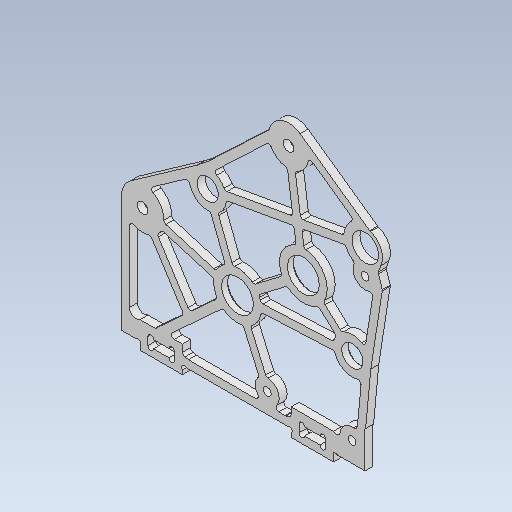
# Autodesk Inventor part: アームフレーム改二
Saved by Autodesk Inventor 2020.2 (Build 242310000, 310)
## iProperties
Created: 2020-02-29
Part Number: アームフレーム改二
Material: アルミニウム 2014-T4
Document SubType Name: Modeling
Designer: aoyam
Density: 2.8 g/cm^3
Appearance: サテン
Mass: 22.4919 g
Surface Area: 98.9037 cm^2
Volume: 8.03281 cm^3
Author: aoyam
Autodesk Inventor part; units mm, degrees
ref_plane "YZ Plane" through (0, 0, 0) normal (1, 0, 0) x (0, 1, 0)
ref_plane "XZ Plane" through (0, 0, 0) normal (0, 1, 0) x (-1, 0, 0)
ref_plane "XY Plane" through (0, 0, 0) normal (0, 0, 1) x (1, 0, 0)
sketch "ギア線図" plane through (0, 0, 0) normal (0, 0, 1) x (1, 0, 0)
  circle A0 centre (11.2246, -29.111) radius 11.1
  circle A1 centre (54.569, -27.2294) radius 20.05
  circle A2 centre (54.569, -27.2294) radius 4
  circle A3 centre (36.0807, -10.2532) radius 11.1
  circle A4 centre (39.569, -43.72) radius 2.05
  circle A5 centre (69.569, -43.72) radius 2.05
  circle A6 centre (72.4026, -13.8541) radius 2.05
  circle A7 centre (39.569, -43.72) radius 15
  circle A8 centre (69.569, -43.72) radius 15
  circle A9 centre (72.4026, -13.8541) radius 15
  circle A10 centre (54.569, -27.2294) radius 5.5 construction
  circle A11 centre (11.2246, -29.111) radius 13 construction
  circle A12 centre (54.569, -27.2294) radius 20.5 construction
  circle A13 centre (36.0807, -10.2532) radius 20.55
  circle A14 centre (36.0807, -10.2532) radius 21.5 construction
  circle A15 centre (36.0807, -10.2532) radius 13 construction
  circle A16 centre (39.569, -43.72) radius 2.5 construction
  circle A17 centre (69.569, -43.72) radius 2.5 construction
  circle A18 centre (72.4026, -13.8541) radius 2.5 construction
  circle A19 centre (11.2246, -29.111) radius 20.1
  circle A20 centre (11.2246, -29.111) radius 22 construction
  line L0 (39.569, -43.72) -> (69.569, -43.72)
  circle A21 centre (0, 0) radius 20.1
  circle A22 centre (0, 0) radius 22 construction
  circle A23 centre (39.569, -43.72) radius 9.5 construction
  circle A24 centre (69.569, -43.72) radius 9.5 construction
  circle A25 centre (72.4026, -13.8541) radius 9.5 construction
  line L1 (39.569, -43.72) -> (33.651, -38.3369)
  line L2 (39.569, -43.72) -> (54.569, -27.2294)
  circle A26 centre (33.651, -38.3369) radius 2.25
  circle A27 centre (54.569, -27.2294) radius 4.55
  line L3 (39.569, -43.72) -> (45.487, -49.103)
  circle A28 centre (45.487, -49.103) radius 1.3
  line L4 (69.569, -43.72) -> (54.569, -27.2294)
  line L5 (54.569, -27.2294) -> (72.4026, -13.8541)
  line L6 (69.569, -43.72) -> (75.487, -38.3369)
  line L7 (69.569, -43.72) -> (63.651, -49.103)
  circle A29 centre (63.651, -49.103) radius 1.3
  circle A30 centre (75.487, -38.3369) radius 1.3
  line L8 (39.569, -43.72) -> (11.2246, -29.111)
  line L9 (77.2027, -20.2541) -> (72.4026, -13.8541)
  circle A31 centre (77.2027, -20.2541) radius 1.3
  circle A32 centre (67.6026, -7.4541) radius 1.3
  point P0 (58.2233, -20.0465)
  point P1 (42.0436, -35)
  point P2 (21.5995, 15.2696)
  point P3 (38.2329, 5.9161)
  point P4 (24.1755, 8.4229)
  point P5 (21.6039, 15.1272)
  point P6 (23.3458, 16.3469)
  point P7 (23.3177, 16.3886)
  dimension "d7" = 22.2
  dimension "d8" = 40.1
  dimension "d9" = 8
  dimension "d11" = 22.2
  dimension "d12" = 4.1
  dimension "d13" = 4.1
  dimension "d14" = 4.1
  dimension "d15" = 30
  dimension "d16" = 30
  dimension "d17" = 30
  dimension "d18" = 11
  dimension "d21" = 26
  dimension "d29" = 41
  dimension "d39" = 22.2921
  dimension "d40" = 22.2921
  dimension "d41" = 22.2921
  dimension "d43" = 41.1
  dimension "d44" = 43
  dimension "d45" = 26
  dimension "d46" = 5
  dimension "d47" = 5
  dimension "d48" = 5
  dimension "d49" = 40.2
  dimension "d50" = 44
  dimension "d53" = 40.2
  dimension "d55" = 44
  dimension "d58" = 19
  dimension "d59" = 19
  dimension "d60" = 19
  dimension "d86" = 8
  dimension "d87" = 4.5
  dimension "d121" = 8
  dimension "d122" = 2.6
  dimension "d123" = 8
  dimension "d124" = 8
  dimension "d125" = 2.6
  dimension "d126" = 2.6
  dimension "d127" = 31.8878
  dimension "d128" = 8
  dimension "d129" = 2.6
  constraints: 33 centre point, 20 coincident, 20 end point, 7 tangent, 5 perpendicular, 3 concentric, 2 horizontal, 1 symmetric about line, 2 other
  measures "d7" diameter of A0
  measures "d8" diameter of A1
  measures "d9" diameter of A2
  measures "d11" diameter of A3
  measures "d12" diameter of A4
  measures "d13" diameter of A5
  measures "d14" diameter of A6
  measures "d15" diameter of A7
  measures "d16" diameter of A8
  measures "d17" diameter of A9
  measures "d18" diameter of A10
  measures "d21" diameter of A11
  measures "d29" diameter of A12
  measures "d39" distance of A4.centre A1.centre
  measures "d40" distance of A5.centre A1.centre
  measures "d41" distance of A6.centre A1.centre
  measures "d43" diameter of A13
  measures "d44" diameter of A14
  measures "d45" diameter of A15
  measures "d46" diameter of A16
  measures "d47" diameter of A17
  measures "d48" diameter of A18
  measures "d49" diameter of A19
  measures "d50" diameter of A20
  measures "d53" diameter of A21
  measures "d55" diameter of A22
  measures "d58" diameter of A23
  measures "d59" diameter of A24
  measures "d60" diameter of A25
  measures "d86" distance of L1.start L1.end
  measures "d87" diameter of A26
  measures "d121" distance of L1.start L3.end
  measures "d122" diameter of A28
  measures "d123" distance of L4.start L6.end
  measures "d124" distance of L7.start L7.end
  measures "d125" diameter of A29
  measures "d126" diameter of A30
  measures "d127" distance of L1.start L8.end
  measures "d128" distance of L9.start L5.end
  measures "d129" diameter of A31
sketch "スケッチ3" plane through (0, 0, 0) normal (0, 0, 1) x (1, 0, 0)
  circle A0 centre (54.569, -27.2294) radius 20.05 construction
  circle A1 centre (39.569, -43.72) radius 2.05 construction
  circle A2 centre (69.569, -43.72) radius 2.05 construction
  circle A3 centre (72.4026, -13.8541) radius 2.05 construction
  circle A4 centre (39.569, -43.72) radius 15 construction
  circle A5 centre (69.569, -43.72) radius 15 construction
  circle A6 centre (72.4026, -13.8541) radius 15 construction
  line L0 (39.569, -43.72) -> (45.487, -49.103)
  line L1 (45.487, -49.103) -> (39.569, -43.72)
  line L2 (39.569, -43.72) -> (33.651, -38.3369)
  line L3 (39.569, -43.72) -> (41.0777, -42.0614)
  circle A7 centre (33.651, -38.3369) radius 1.3
  circle A8 centre (45.487, -49.103) radius 1.3
  line L4 (69.569, -43.72) -> (68.0603, -42.0614)
  line L5 (69.569, -43.72) -> (75.487, -38.3369)
  line L6 (69.569, -43.72) -> (63.651, -49.103)
  circle A9 centre (63.651, -49.103) radius 1.3
  circle A10 centre (75.487, -38.3369) radius 1.3
  line L7 (72.4026, -13.8541) -> (70.609, -15.1993)
  line L8 (67.6026, -7.4541) -> (72.4026, -13.8541)
  line L9 (72.4026, -13.8541) -> (77.2027, -20.2541)
  circle A11 centre (67.6026, -7.4541) radius 1.3
  circle A12 centre (77.2027, -20.2541) radius 1.3
  circle A13 centre (39.569, -43.72) radius 5
  circle A14 centre (69.569, -43.72) radius 5
  circle A15 centre (72.4026, -13.8541) radius 5
  circle A16 centre (54.569, -27.2294) radius 4
  circle A17 centre (36.0807, -10.2532) radius 11.1 construction
  line L10 (87.4026, -58.72) -> (21.3486, -58.72)
  line L11 (87.4026, 3.1749) -> (87.4026, -58.72)
  circle A18 centre (36.0807, -10.2532) radius 6
  circle A19 centre (23.1948, 12.8161) radius 1.5
  circle A20 centre (59.3303, 1.1874) radius 1.5
  circle A21 centre (11.2246, -29.111) radius 6
  circle A22 centre (14.4482, -54.9706) radius 1.5
  line L12 (87.4026, 3.1749) -> (31.1389, 3.1749)
  line L13 (31.1389, 3.1749) -> (25.7575, 16.2256)
  line L14 (26.6296, -46.3454) -> (10.2913, -53.0824)
  line L15 (10.2913, -53.0824) -> (10.2913, -58.72)
  line L16 (10.2913, -58.72) -> (21.3486, -58.72)
  line L17 (26.6296, -46.3454) -> (26.6296, -10.2532)
  line L18 (26.6296, -10.2532) -> (18.7982, 13.9762)
  line L19 (18.7982, 13.9762) -> (25.7575, 16.2256)
  circle A23 centre (36.0807, -10.2532) radius 13 projected
  circle A24 centre (36.0807, -10.2532) radius 14
  circle A25 centre (36.0807, -10.2532) radius 17
  line L20 (50.0807, -10.2532) -> (50.0807, 3.1749)
  line L21 (26.6296, -24.2532) -> (36.0807, -24.2532)
  circle A26 centre (33.651, -38.3369) radius 2
  point P0 (0, 0)
  point P1 (0, 0)
  point P2 (30.1122, 5.6646)
  point P3 (23.0867, 0.7083)
  point P4 (26.6296, -24.3839)
  point P5 (46.5059, 3.1749)
  point P6 (40.0412, 3.1749)
  point P7 (26.6296, -20.5817)
  dimension "d61" = 8
  dimension "d62" = 8
  dimension "d63" = 2.6
  dimension "d64" = 2.6
  dimension "d65" = 8
  dimension "d66" = 8
  dimension "d67" = 2.6
  dimension "d68" = 2.6
  dimension "d69" = 8
  dimension "d70" = 8
  dimension "d71" = 2.6
  dimension "d72" = 2.6
  dimension "d73" = 10
  dimension "d74" = 10
  dimension "d75" = 10
  dimension "d76" = 8
  dimension "d79" = 12
  dimension "d82" = 26
  dimension "d83" = 1
  dimension "d84" = 3
  dimension "d85" = 4
  dimension "d98" = 12
  constraints: 44 end point, 18 centre point, 13 coincident, 8 perpendicular, 5 point on circle, 3 horizontal, 3 line through centre, 3 point on line, 2 collinear, 2 tangent, 2 vertical
  measures "d61" distance of L0.start L0.end
  measures "d62" distance of L0.start L2.end
  measures "d63" diameter of A7
  measures "d64" diameter of A8
  measures "d65" distance of L4.start L5.end
  measures "d66" distance of L4.start L6.end
  measures "d67" diameter of A9
  measures "d68" diameter of A10
  measures "d69" distance of L8.start L8.end
  measures "d70" distance of L8.end L9.end
  measures "d71" diameter of A11
  measures "d72" diameter of A12
  measures "d73" diameter of A13
  measures "d74" diameter of A14
  measures "d75" diameter of A15
  measures "d76" diameter of A16
  measures "d79" diameter of A18
  measures "d82" diameter of A23
  measures "d83" radial gap between concentric circles of A23 A24
  measures "d84" radial gap between concentric circles of A24 A25
  measures "d85" diameter of A26
  measures "d98" diameter of A21
sketch "スケッチ6" plane through (0, 0, 0) normal (0, 0, 1) x (1, 0, 0)
  circle A0 centre (36.0807, -10.2532) radius 6 projected
  circle A1 centre (11.2246, -29.111) radius 6 projected
  circle A2 centre (54.569, -27.2294) radius 4 projected
  circle A3 centre (14.4482, -54.9706) radius 1.5 projected
  circle A4 centre (59.3303, 1.1874) radius 1.5 projected
  line L0 (-26.5518, -24.6836) -> (-26.5518, -65.4706)
  line L1 (-26.5518, -65.4706) -> (62.634, -65.4706)
  line L2 (62.7829, 5.6168) -> (32.1759, 5.6168)
  line L3 (-26.5518, -24.6836) -> (-26.5518, 11.7202)
  line L4 (-26.5518, 11.7202) -> (32.1759, 5.6168)
  circle A5 centre (9.9716, -0.138) radius 1.5
  line L5 (14.4482, -54.9706) -> (22.4482, -54.9706)
  circle A6 centre (22.4482, -54.9706) radius 1.5
  circle A7 centre (0, 0) radius 4.025
  circle A8 centre (0, 0) radius 6.025
  circle A9 centre (54.4482, -54.9706) radius 1.5
  circle A10 centre (39.569, -43.72) radius 15 projected
  circle A11 centre (69.569, -43.72) radius 15 projected
  circle A12 centre (34.7829, 12.7101) radius 1.5
  circle A13 centre (34.7829, 12.7101) radius 3
  line L6 (10.3237, 7.8878) -> (33.8527, 15.5623)
  line L7 (45.0708, 5.6168) -> (37.029, 14.6989)
  line L8 (62.7829, 5.6168) -> (62.7829, 15.7101)
  line L9 (62.7829, 15.7101) -> (34.7829, 15.7101)
  circle A14 centre (59.4482, 10.5294) radius 5.025
  line L10 (54.4482, -54.9706) -> (54.4482, -65.4706)
  line L11 (36.0807, -10.2532) -> (30.5138, 29.3575)
  circle A15 centre (30.5138, 29.3575) radius 2
  circle A16 centre (30.5138, 29.3575) radius 7.5
  line L12 (18.8335, 10.6635) -> (23.1806, 30.9304)
  line L13 (34.8461, 35.4797) -> (62.7829, 15.7101)
  circle A17 centre (59.4482, 10.5294) radius 1.3831
  circle A18 centre (59.4482, 10.5294) radius 6.525
  line L14 (33.651, -38.3369) -> (45.487, -49.103) construction
  line L15 (62.7829, 15.7101) -> (65.8383, 5.6859)
  line L16 (65.8383, 5.6859) -> (65.8383, -65.4706)
  line L17 (65.8383, -65.4706) -> (62.634, -65.4706)
  line L18 (63.651, -49.103) -> (75.422, -38.396) construction
  circle A19 centre (33.651, -38.3369) radius 3.25
  circle A20 centre (45.487, -49.103) radius 3.25
  circle A21 centre (63.651, -49.103) radius 3.25
  circle A22 centre (75.487, -38.3369) radius 3.25
  circle A23 centre (67.6026, -7.4541) radius 3.25
  circle A24 centre (77.2027, -20.2541) radius 3.25
  line L19 (20, -56.4706) -> (25.0061, -56.4706)
  circle A25 centre (39.569, -43.72) radius 2.75
  circle A26 centre (69.569, -43.72) radius 2.75
  circle A27 centre (72.4026, -13.8541) radius 2.75
  line L20 (-22.5518, -62.4706) -> (-12.5518, -62.4706)
  line L21 (-12.5518, -62.4706) -> (-12.5518, -59.4706)
  line L22 (-12.5518, -59.4706) -> (-22.5518, -59.4706)
  line L23 (-22.5518, -59.4706) -> (-22.5518, -62.4706)
  line L24 (44.4482, -59.4706) -> (34.4482, -59.4706)
  line L25 (34.4482, -59.4706) -> (34.4482, -62.4706)
  line L26 (34.4482, -62.4706) -> (39.4482, -62.4706)
  line L27 (44.4482, -62.4706) -> (44.4482, -59.4706)
  line L28 (39.4482, -62.4706) -> (44.4482, -62.4706)
  line L29 (65.8383, -62.4706) -> (-26.5518, -62.4706)
  line L30 (-25.5518, -65.4706) -> (-9.5518, -65.4706)
  line L31 (-9.5518, -65.4706) -> (-9.5518, -54.0997)
  line L32 (-9.5518, -54.0997) -> (-25.5518, -54.0997)
  line L33 (-25.5518, -54.0997) -> (-25.5518, -65.4706)
  line L34 (47.4482, -65.4706) -> (31.4482, -65.4706)
  line L35 (31.4482, -65.4706) -> (31.4482, -56.8819)
  line L36 (31.4482, -56.8819) -> (47.4482, -56.8819)
  line L37 (47.4482, -56.8819) -> (47.4482, -65.4706)
  circle A28 centre (-8.8412, -63.1813) radius 1.005
  line L38 (48.1588, -63.1813) -> (47.4482, -62.4706)
  circle A29 centre (48.1588, -63.1813) radius 1.005
  circle A30 centre (30.8584, -63.1813) radius 1.005
  line L39 (-8.8412, -63.1813) -> (-9.5518, -62.4706)
  line L40 (-17.5518, -54.0997) -> (-17.5518, -59.4706)
  circle A31 centre (-26.2625, -63.1813) radius 1.005
  line L41 (-26.5518, 11.7202) -> (-32.5518, 11.7202)
  line L42 (-32.5518, 11.7202) -> (-32.5518, -62.4706)
  line L43 (-32.5518, -62.4706) -> (-26.5518, -62.4706)
  line L44 (-26.5518, -62.4706) -> (-26.5518, 11.7202)
  line L45 (0, 8.9607) -> (-32.5518, 0)
  line L46 (22.4482, -54.9706) -> (54.4482, -54.9706)
  line L47 (63.651, -49.103) -> (69.5365, -43.7495)
  line L48 (69.5365, -43.7495) -> (75.487, -38.3369)
  line L49 (65.8383, 5.6859) -> (59.3303, -13.8541)
  line L50 (59.3303, -13.8541) -> (59.3303, -65.4706)
  circle A32 centre (-21.5018, -59.4706) radius 1.05
  circle A33 centre (-21.5018, -62.4706) radius 1.05
  line L51 (-22.5518, -62.4706) -> (-21.5018, -62.4706)
  circle A34 centre (-13.6018, -59.4706) radius 1.05
  circle A35 centre (-13.6018, -62.4706) radius 1.05
  line L52 (-13.6018, -62.4706) -> (-12.5518, -62.4706)
  line L53 (-12.5518, -59.4706) -> (-13.6018, -59.4706)
  circle A36 centre (35.4982, -59.4706) radius 1.05
  circle A37 centre (35.4982, -62.4706) radius 1.05
  circle A38 centre (43.3982, -59.4706) radius 1.05
  circle A39 centre (43.3982, -62.4706) radius 1.05
  line L54 (59.3303, -48.7583) -> (65.8383, -42.4712)
  circle A40 centre (59.4482, 10.5294) radius 7.525
  line L55 (64.3298, 4.8026) -> (65.8383, 0)
  line L56 (0, 8.9607) -> (23.1806, 30.9304)
  line L57 (65.2638, 7.5706) -> (64.3298, 4.8026)
  point P0 (57.1451, 15.7101)
  point P1 (61.5154, 15.7101)
  point P2 (61.2364, 16.8045)
  point P3 (65.2437, 7.5808)
  point P4 (62.7829, 14.2884)
  point P5 (62.7829, 6.7704)
  point P6 (31.4482, -62.4706)
  point P7 (77.569, -62.4706)
  point P8 (-25.5518, -62.4706)
  point P9 (-9.5518, -65.4706)
  point P10 (-26.5518, -62.2188)
  point P11 (-25.5518, -63.8919)
  point P12 (-9.5518, -63.8919)
  point P13 (-8.1305, -62.4706)
  point P14 (30.1477, -62.4706)
  point P15 (31.4482, -63.995)
  point P16 (47.4482, -63.8919)
  point P17 (48.8695, -62.4706)
  point P18 (-26.9731, -62.4706)
  point P19 (-26.5518, 1.6517)
  point P20 (59.3303, -62.4706)
  point P21 (65.8383, -10.1835)
  point P22 (65.8383, -4.7247)
  point P23 (34.4482, -59.4706)
  point P24 (34.4482, -62.4706)
  point P25 (44.4482, -59.4706)
  point P26 (44.4482, -62.4706)
  point P27 (34.4482, -62.4706)
  point P28 (34.4482, -59.4706)
  point P29 (42.3482, -59.4706)
  point P30 (44.4482, -59.4706)
  point P31 (44.4482, -62.4706)
  point P32 (42.3482, -62.4706)
  point P33 (36.5482, -62.4706)
  point P34 (-22.5518, -60.9857)
  point P35 (-22.5518, -60.9556)
  point P36 (-20.4518, -59.4706)
  point P37 (-14.6518, -59.4706)
  point P38 (-12.5518, -60.9558)
  point P39 (-12.5518, -60.9839)
  point P40 (-14.6518, -62.4706)
  point P41 (-20.4518, -62.4706)
  point P42 (36.5482, -59.4706)
  point P43 (65.6576, 6.2786)
  point P44 (59.4703, 18.0543)
  point P45 (49.4898, -54.9706)
  point P46 (29.6482, -54.9706)
  point P47 (0.2203, 8.9379)
  point P48 (64.7988, 3.2895)
  point P49 (65.8383, 4.1881)
  point P50 (60.7654, 1.6238)
  point P51 (57.9066, 1.6598)
  point P52 (60.5054, 5.6168)
  point P53 (58.3909, 5.6168)
  point P54 (62.7829, 10.8919)
  point P55 (62.7829, 10.1668)
  dimension "d172" = 2.01
  dimension "d175" = 2.01
  dimension "d239" = 2.1
  dimension "d241" = 2.1
  dimension "d243" = 2.1
  dimension "d244" = 2.1
  dimension "d101" = 3
  dimension "d102" = 28
  dimension "d103" = 29
  dimension "d104" = 8
  dimension "d105" = 3
  dimension "d106" = 8.05
  dimension "d107" = 12.05
  dimension "d118" = 3
  dimension "d130" = 3
  dimension "d131" = 48
  dimension "d133" = 23
  dimension "d134" = 6
  dimension "d136" = 10.05
  dimension "d137" = 10.5
  dimension "d140" = 40
  dimension "d141" = 4
  dimension "d142" = 15
  dimension "d144" = 98
  dimension "d146" = 1.5
  dimension "d149" = 6.5
  dimension "d150" = 6.5
  dimension "d151" = 6.5
  dimension "d152" = 6.5
  dimension "d153" = 6.5
  dimension "d154" = 6.5
  dimension "d156" = 9
  dimension "d157" = 5.5
  dimension "d158" = 5.5
  dimension "d159" = 5.5
  dimension "d160" = 41
  dimension "d161" = 10
  dimension "d162" = 3
  dimension "d163" = 4
  dimension "d164" = 3
  dimension "d165" = 10
  dimension "d166" = 3
  dimension "d167" = 3
  dimension "d168" = 16
  dimension "d169" = 3
  dimension "d170" = 16
  dimension "d171" = 3
  dimension "d173" = 3
  dimension "d174" = 45
  dimension "d176" = 45
  dimension "d185" = 6
  dimension "d186" = 32
  dimension "d187" = 8
  dimension "d188" = 8
  dimension "d189" = 41
  dimension "d249" = 57
  dimension "d262" = 2.5
  dimension "d266" = 28
  dimension "d313" = 73
  dimension "d315" = 12
  constraints: 120 end point, 22 centre point, 20 point on line, 16 coincident, 16 horizontal, 11 parallel, 11 vertical, 7 perpendicular, 7 tangent, 5 point on circle, 4 midpoint, 3 collinear, 1 symmetric about line, 47 other
  measures "d101" diameter of A5
  measures "d102" distance of A5.centre L11.start
  measures "d103" distance of A5.centre A1.centre
  measures "d104" distance of L5.start L5.end
  measures "d105" diameter of A6
  measures "d106" diameter of A7
  measures "d107" diameter of A8
  measures "d118" diameter of A9
  measures "d130" diameter of A12
  measures "d131" distance of A12.centre A1.centre
  measures "d133" distance of L11.start A12.centre
  measures "d134" diameter of A13
  measures "d136" diameter of A14
  measures "d137" distance of L10.start L10.end
  measures "d140" distance of L11.start L11.end
  measures "d141" diameter of A15
  measures "d142" diameter of A16
  measures "d144" angle of L11 L9
  measures "d149" diameter of A19
  measures "d150" diameter of A20
  measures "d151" diameter of A21
  measures "d152" diameter of A22
  measures "d153" diameter of A23
  measures "d154" diameter of A24
  measures "d156" distance between parallel lines of L1 L19
  measures "d157" diameter of A25
  measures "d158" diameter of A26
  measures "d159" diameter of A27
  measures "d160" distance from line of L0 L5.start
  measures "d161" distance of L22.end L21.end
  measures "d162" distance of L21.end L20.end
  measures "d163" distance between parallel lines of L23 L0
  measures "d164" distance between parallel lines of L1 L20
  measures "d165" distance of L27.start L25.end
  measures "d166" distance of L25.end L24.end
  measures "d167" distance between parallel lines of L28 L17
  measures "d168" distance of L31.end L32.end
  measures "d169" distance between parallel lines of L31 L21
  measures "d170" distance of L35.end L36.end
  measures "d171" distance between parallel lines of L37 L27
  measures "d173" distance between parallel lines of L34 L29
  measures "d174" angle of L37 L38
  measures "d176" angle of L39 L29
  measures "d185" distance of L43.end L42.end
  measures "d186" distance of L46.start L10.start
  measures "d187" distance of A26.centre L48.end
  measures "d188" distance of L47.start A26.centre
  measures "d189" distance between parallel lines of L35 L31
  measures "d249" distance of point (-21.502, -59.471) point (35.498, -59.471)
  measures "d266" distance of L8.end L9.end
  measures "d313" distance from line of L29 A14.centre
  measures "d315" distance from line of A14.centre L37
extrude "押し出し3" add sketch "スケッチ6" along normal blind 3 contours A3 | L3 L45 L4 L2 A40 L55 L49 L50 A11 A10 L36 L35 A30 L29 A28 L31 L32 L33 A31 L0 | L0 A31 L43 L42 L45 L3 | L33 L32 L40 L22 A32 L23 L29 | L29 A33 L20 A35 A28 L31 L1 L33 A31 | L56 L12 L6 L4 | L6 L11 A13 L2 L4 | A16 | A16 L11 L6 L12 | L32 L31 L29 L21 A34 L22 L40 | L13 A40 L9 A13 L6 L11 A16 | L11 A13 L7 L2 | L6 A13 L11 | L13 A18 L9 A40 | L35 A30 L29 A37 L26 L28 A39 A29 L37 L1 | L7 A13 L9 A40 L2 | L11 A13 | A13 L11 | A18 L15 A14 L13 | L13 L9 A18 | L9 A18 L2 A40 | L2 A18 L57 A40 | L15 A14 L8 | L8 A14 L2 A18 L9 | A29 L37 | L2 A14 L8 L15 A18 | L35 L36 A10 L37 L29 L27 A38 L24 A36 L25 A30 | L29 A29 L37 L36 A10 L46 A9 L10 | L10 A9 L46 A10 A11 L50 L29 | L55 L16 A23 A11 L50 L49 | L8 L2 A14 | L16 A23 | L36 A10 | A10 L46 L36 | A11 L50 | A11 L16 L54 L50 | A10 L46 | A5 | A8 | A12 picked at (62.8591, 14.6903) picked at (62.5531, 6.2147) picked at (65.3431, -7.4541)
sketch "スケッチ7" plane through (0, 0, 0) normal (0, 0, -1) x (-1, 0, 0)
  circle A0 centre (-54.569, -27.2294) radius 4 projected
  circle A1 centre (-36.0807, -10.2532) radius 6 projected
  circle A2 centre (-11.2246, -29.111) radius 6 projected
  circle A3 centre (-54.569, -27.2294) radius 4.6
  circle A4 centre (-36.0807, -10.2532) radius 6.8
  circle A5 centre (-11.2246, -29.111) radius 6.8
  point P0 (0, 0)
  dimension "d90" = 0.6
  dimension "d92" = 0.8
  dimension "d93" = 0.8
  constraints: 3 centre point
  measures "d90" radial gap between concentric circles of A0 A3
  measures "d92" radial gap between concentric circles of A1 A4
  measures "d93" radial gap between concentric circles of A2 A5
extrude "押し出し4" cut sketch "スケッチ7" against normal blind 0.6 contours A3
extrude "押し出し5" cut sketch "スケッチ7" against normal blind 0.8 contours A4 | A5
sketch "スケッチ11" plane through (0, 0, 0) normal (0, 0, -1) x (-1, 0, 0)
  circle A0 centre (-22.4482, -54.9706) radius 1.5 projected
  circle A1 centre (-22.4482, -54.9706) radius 3
  circle A2 centre (-59.3303, 1.1874) radius 1.5 projected
  circle A3 centre (-59.3303, 1.1874) radius 3
  point P0 (0, 0)
  point P1 (-60.8303, 1.1874)
  point P2 (-60.8303, 1.1874)
  dimension "d111" = 6
  dimension "d114" = 6
  constraints: 2 centre point, 2 coincident
  measures "d111" diameter of A1
  measures "d114" diameter of A3
extrude "押し出し7" cut sketch "スケッチ11" against normal blind 0.4 contours A1 | A2 | A3
sketch "スケッチ12" plane through (0, 0, 0) normal (0, 0, -1) x (-1, 0, 0)
  circle A0 centre (24.5518, -18.4706) radius 2
  arc A1 (16.539, -4.2191) -> (53.857, -2.4442) centre (33.3581, 35.3552) ccw construction
  line L0 (12.562, -4.4082) -> (16.539, -4.2191) construction
  circle A2 centre (24.5518, -18.4706) radius 4
  line L1 (20.4518, -59.4706) -> (14.6518, -59.4706) projected
  line L2 (22.5518, -62.4706) -> (22.5518, -59.4706) projected
  point P0 (0, 0)
  point P1 (12.5518, -59.4706)
  dimension "d178" = 4
  dimension "d181" = 8
  dimension "d182" = 41
  dimension "d184" = 2
  constraints: 2 centre point, 1 coincident
  measures "d178" diameter of A0
  measures "d181" diameter of A2
  measures "d182" distance from line of A0.centre L1
  measures "d184" distance from line of A0.centre L2
extrude "押し出し8" cut sketch "スケッチ12" against normal blind 10 contours A0
sketch "スケッチ13" plane through (0, 0, 3) normal (0, 0, 1) x (1, 0, 0)
  circle A0 centre (-24.5518, -18.4706) radius 2
  line L0 (-9.5518, -65.4706) -> (-9.5518, -63.8919) projected
  arc A1 (-8.1305, -62.4706) -> (-9.5518, -63.8919) centre (-8.8412, -63.1813) ccw projected
  line L1 (-8.1305, -62.4706) -> (30.1477, -62.4706) projected
  arc A2 (31.4482, -63.995) -> (30.1477, -62.4706) centre (30.8584, -63.1813) ccw projected
  line L2 (31.4482, -63.995) -> (31.4482, -65.4706) projected
  line L3 (31.4482, -65.4706) -> (47.4482, -65.4706) projected
  line L4 (47.4482, -65.4706) -> (47.4482, -62.4706) projected
  arc A3 (48.8695, -62.4706) -> (47.4482, -62.4706) centre (48.1588, -63.1813) ccw projected
  line L5 (48.8695, -62.4706) -> (59.3303, -62.4706) projected
  line L6 (65.8383, -42.4712) -> (65.8383, 0) projected
  line L7 (61.2364, 16.8045) -> (34.8461, 35.4797) projected
  arc A4 (34.8461, 35.4797) -> (23.1806, 30.9304) centre (30.5138, 29.3575) ccw projected
  line L8 (0, 8.9607) -> (-32.5518, 0) projected
  line L9 (-32.5518, 0) -> (-32.5518, -62.4706) projected
  line L10 (-32.5518, -62.4706) -> (-26.9731, -62.4706) projected
  arc A5 (-25.5518, -63.8919) -> (-26.9731, -62.4706) centre (-26.2625, -63.1813) ccw projected
  line L11 (-25.5518, -63.8919) -> (-25.5518, -65.4706) projected
  line L12 (-25.5518, -65.4706) -> (-9.5518, -65.4706) projected
  circle A6 centre (54.4482, -54.9706) radius 1.5 projected
  circle A7 centre (22.4482, -54.9706) radius 1.5 projected
  circle A8 centre (36.0807, -10.2532) radius 6 projected
  circle A9 centre (59.3303, 1.1874) radius 1.5 projected
  circle A10 centre (54.569, -27.2294) radius 4 projected
  circle A11 centre (11.2246, -29.111) radius 6 projected
  circle A12 centre (0, 0) radius 4.025 projected
  circle A13 centre (30.5138, 29.3575) radius 2 projected
  line L13 (59.3303, -62.4706) -> (59.3303, -48.7583) projected
  line L14 (59.3303, -48.7583) -> (65.8383, -42.4712) projected
  line L15 (23.1806, 30.9304) -> (0, 8.9607) projected
  line L16 (-29.5518, -2.2858) -> (1.5193, 6.2674)
  line L17 (1.5193, 6.2674) -> (26.0155, 29.484)
  arc A14 (33.1132, 33.0308) -> (26.0155, 29.484) centre (30.5138, 29.3575) ccw
  line L18 (33.1132, 33.0308) -> (57.9105, 15.4829)
  arc A15 (60.9658, 5.5696) -> (57.9105, 15.4829) centre (59.4482, 10.5294) ccw
  line L19 (60.9658, 5.5696) -> (62.8383, -0.438)
  line L20 (62.8383, -0.438) -> (62.8383, -41.1981)
  line L21 (62.8383, -41.1981) -> (56.3303, -47.4852)
  line L22 (56.3303, -47.4852) -> (56.3303, -59.4706)
  line L23 (56.3303, -59.4706) -> (49.6659, -59.4706)
  arc A16 (49.6659, -59.4706) -> (44.4482, -61.6742) centre (48.1588, -63.1813) ccw
  line L24 (44.4482, -61.6742) -> (44.4482, -62.4706)
  line L25 (44.4482, -62.4706) -> (34.7998, -62.4706)
  arc A17 (34.7998, -62.4706) -> (29.3513, -59.4706) centre (30.8584, -63.1813) ccw
  line L26 (29.3513, -59.4706) -> (-7.3341, -59.4706)
  arc A18 (-7.3341, -59.4706) -> (-12.7826, -62.4706) centre (-8.8412, -63.1813) ccw
  line L27 (-12.7826, -62.4706) -> (-22.321, -62.4706)
  arc A19 (-22.321, -62.4706) -> (-29.5518, -60.8965) centre (-26.2625, -63.1813) ccw
  line L28 (-29.5518, -60.8965) -> (-29.5518, -2.2858)
  circle A20 centre (30.5138, 29.3575) radius 7.5
  circle A21 centre (59.4482, 10.5294) radius 8.0025
  circle A22 centre (36.0807, -10.2532) radius 9
  circle A23 centre (11.2246, -29.111) radius 9
  circle A24 centre (54.569, -27.2294) radius 7
  circle A25 centre (22.4482, -54.9706) radius 4.5
  circle A26 centre (54.4482, -54.9706) radius 4.5
  line L29 (-9.5518, -65.4706) -> (-25.5518, -65.4706)
  line L30 (-25.5518, -65.4706) -> (-25.5518, -55.4706)
  line L31 (-25.5518, -55.4706) -> (-9.5518, -55.4706)
  line L32 (-9.5518, -55.4706) -> (-9.5518, -65.4706)
  line L33 (47.4482, -65.4706) -> (31.4482, -65.4706)
  line L34 (31.4482, -65.4706) -> (31.4482, -55.4706)
  line L35 (31.4482, -55.4706) -> (47.4482, -55.4706)
  line L36 (47.4482, -55.4706) -> (47.4482, -65.4706)
  line L37 (-24.5518, -18.4706) -> (11.2246, -29.111) construction
  line L38 (-24.9794, -19.9084) -> (10.797, -30.5487)
  line L39 (11.6522, -27.6732) -> (-24.1242, -17.0329)
  arc A27 (-24.1242, -17.0329) -> (-24.9794, -19.9084) centre (-24.5518, -18.4706) ccw
  arc A28 (10.797, -30.5487) -> (11.6522, -27.6732) centre (11.2246, -29.111) ccw
  line L40 (0, 0) -> (11.2246, -29.111) construction
  line L41 (-1.3996, -0.5396) -> (9.825, -29.6506)
  line L42 (12.6242, -28.5713) -> (1.3996, 0.5396)
  arc A29 (1.3996, 0.5396) -> (-1.3996, -0.5396) centre (0, 0) ccw
  arc A30 (9.825, -29.6506) -> (12.6242, -28.5713) centre (11.2246, -29.111) ccw
  line L43 (36.0807, -10.2532) -> (11.2246, -29.111) construction
  line L44 (35.1741, -9.0582) -> (10.318, -27.916)
  line L45 (12.1312, -30.306) -> (36.9873, -11.4482)
  arc A31 (36.9873, -11.4482) -> (35.1741, -9.0582) centre (36.0807, -10.2532) ccw
  arc A32 (10.318, -27.916) -> (12.1312, -30.306) centre (11.2246, -29.111) ccw
  line L46 (54.569, -27.2294) -> (36.0807, -10.2532) construction
  line L47 (55.5835, -26.1245) -> (37.0952, -9.1483)
  line L48 (35.0662, -11.3581) -> (53.5545, -28.3343)
  arc A33 (53.5545, -28.3343) -> (55.5835, -26.1245) centre (54.569, -27.2294) ccw
  arc A34 (37.0952, -9.1483) -> (35.0662, -11.3581) centre (36.0807, -10.2532) ccw
  circle A35 centre (-24.5518, -18.4706) radius 2 projected
  line L49 (30.5138, 29.3575) -> (36.0807, -10.2532) construction
  line L50 (29.0284, 29.1487) -> (34.5953, -10.462)
  line L51 (37.5661, -10.0445) -> (31.9992, 29.5663)
  arc A36 (31.9992, 29.5663) -> (29.0284, 29.1487) centre (30.5138, 29.3575) ccw
  arc A37 (34.5953, -10.462) -> (37.5661, -10.0445) centre (36.0807, -10.2532) ccw
  line L52 (0, 0) -> (59.4482, 10.5294) construction
  line L53 (0.2616, -1.477) -> (59.7098, 9.0524)
  line L54 (59.1866, 12.0064) -> (-0.2616, 1.477)
  arc A38 (-0.2616, 1.477) -> (0.2616, -1.477) centre (0, 0) ccw
  arc A39 (59.7098, 9.0524) -> (59.1866, 12.0064) centre (59.4482, 10.5294) ccw
  circle A40 centre (59.3303, 1.1874) radius 4.5
  line L55 (67.3549, 9.2952) -> (61.4853, -28.309)
  line L56 (61.5377, -27.8906) -> (58.9281, -55.3957)
  line L57 (22.4482, -54.9706) -> (11.2246, -29.111) construction
  line L58 (23.8242, -54.3734) -> (12.6006, -28.5138)
  line L59 (9.8486, -29.7082) -> (21.0722, -55.5678)
  arc A41 (21.0722, -55.5678) -> (23.8242, -54.3734) centre (22.4482, -54.9706) ccw
  arc A42 (12.6006, -28.5138) -> (9.8486, -29.7082) centre (11.2246, -29.111) ccw
  line L60 (11.2246, -29.111) -> (-17.5518, -55.4706) construction
  line L61 (10.2114, -28.0049) -> (-18.565, -54.3645)
  line L62 (-16.5386, -56.5767) -> (12.2378, -30.2171)
  arc A43 (12.2378, -30.2171) -> (10.2114, -28.0049) centre (11.2246, -29.111) ccw
  arc A44 (-18.565, -54.3645) -> (-16.5386, -56.5767) centre (-17.5518, -55.4706) ccw
  line L63 (-24.5518, -18.4706) -> (-7.0912, -45.8885) construction
  line L64 (-25.8171, -19.2764) -> (-8.3564, -46.6943)
  line L65 (-5.826, -45.0828) -> (-23.2866, -17.6649)
  arc A45 (-23.2866, -17.6649) -> (-25.8171, -19.2764) centre (-24.5518, -18.4706) ccw
  arc A46 (-8.3564, -46.6943) -> (-5.826, -45.0828) centre (-7.0912, -45.8885) ccw
  line L66 (58.5511, -27.6072) -> (55.9415, -55.1123)
  line L67 (64.5289, 10.6426) -> (58.5586, -27.6066)
  circle A47 centre (48.4774, -54.3794) radius 1.5
  circle A48 centre (26.7956, -58.4206) radius 1.05
  circle A49 centre (18.1008, -58.4206) radius 1.05
  circle A50 centre (-27.0518, -53.4706) radius 2.5
  circle A51 centre (-24.5518, -18.4706) radius 8
  circle A52 centre (0, 0) radius 7.025
  line L68 (-29.156, -11.9283) -> (-4.043, 5.745)
  line L69 (-27.4241, -14.3779) -> (-2.3118, 3.2949)
  line L70 (0, 8.9607) -> (-4.043, 5.745)
  line L71 (11.2246, -29.111) -> (54.569, -27.2294) construction
  line L72 (11.2897, -30.6096) -> (54.6341, -28.728)
  line L73 (54.504, -25.7308) -> (11.1595, -27.6124)
  arc A53 (11.1595, -27.6124) -> (11.2897, -30.6096) centre (11.2246, -29.111) ccw
  arc A54 (54.6341, -28.728) -> (54.504, -25.7308) centre (54.569, -27.2294) ccw
  line L74 (65.8383, 0) -> (64.3298, 4.8026) projected
  arc A55 (65.2638, 7.5706) -> (61.2364, 16.8045) centre (59.4482, 10.5294) ccw projected
  line L75 (64.3298, 4.8026) -> (65.2638, 7.5706) projected
  point P0 (-32.5518, -22.0997)
  point P1 (-6.6636, -23.7908)
  point P2 (5.6123, -14.5555)
  point P3 (23.6526, -19.6821)
  point P4 (45.3249, -18.7413)
  point P5 (33.2972, 9.5521)
  point P6 (29.7241, 5.2647)
  point P7 (16.8364, -42.0408)
  point P8 (-3.1636, -42.2908)
  point P9 (-15.8215, -32.1796)
  point P10 (35.0674, 7.7344)
  point P11 (51.4464, 10.6354)
  point P12 (55.2677, 17.3531)
  point P13 (38.0109, 29.5649)
  point P14 (33.0219, 22.2893)
  point P15 (32.1115, 7.2109)
  point P16 (30.0511, 21.8718)
  point P17 (23.3941, 26.9995)
  point P18 (32.5293, 4.2382)
  point P19 (9.4316, -20.2914)
  point P20 (17.3877, -22.5523)
  point P21 (28.1043, -14.4219)
  point P22 (33.3602, -1.6742)
  point P23 (59.4071, -22.1705)
  point P24 (62.5647, -1.9413)
  point P25 (55.5088, 3.5636)
  point P26 (51.9696, 7.6814)
  point P27 (35.4852, 4.7617)
  point P28 (36.3311, -1.2567)
  point P29 (43.6318, -15.1503)
  point P30 (50.5472, -21.5001)
  point P31 (26.7956, -59.4706)
  point P32 (31.4482, -59.2199)
  point P33 (49.9701, -54.5272)
  point P34 (56.3303, -50.8831)
  point P35 (56.6989, -47.1291)
  point P36 (58.0085, -33.3261)
  point P37 (48.5182, -23.7099)
  point P38 (41.6027, -17.36)
  point P39 (29.9176, -16.8119)
  point P40 (19.201, -24.9423)
  point P41 (16.1337, -36.6542)
  point P42 (22.135, -50.4815)
  point P43 (25.9731, -57.7679)
  point P44 (-22.576, -18.7807)
  point P45 (-6.7862, -43.575)
  point P46 (3.6677, -33.999)
  point P47 (2.2911, -28.019)
  point P48 (-23.7115, -20.2855)
  point P49 (18.9232, -57.7679)
  point P50 (19.383, -51.676)
  point P51 (13.3817, -37.8486)
  point P52 (5.6941, -36.2112)
  point P53 (-15.3311, -55.4706)
  point P54 (-9.5518, -59.2398)
  point P55 (18.1008, -59.4706)
  point P56 (-19.0518, -55.4706)
  point P57 (-9.0325, -45.6326)
  point P58 (-25.1065, -20.3922)
  point P59 (-29.5518, -24.7156)
  point P60 (-29.5518, -53.4706)
  point P61 (-22.8562, -17.41)
  point P62 (3.1463, -25.1435)
  point P63 (6.6325, -21.3707)
  point P64 (-21.1285, -21.0537)
  point P65 (-6.078, -46.9946)
  point P66 (8.7272, -26.8033)
  point P67 (-17.4474, -22.1485)
  point P68 (-19.0656, -24.2931)
  point P69 (-7.025, -0.022)
  point P70 (-22.3223, -10.7876)
  point P71 (-16.5922, -19.273)
  point P72 (1.0695, -6.9431)
  point P73 (2.0091, 6.7316)
  point P74 (6.4962, 2.6739)
  point P75 (7.0194, -0.2801)
  point P76 (3.8686, -5.8638)
  point P77 (59.5808, -48.5163)
  point P78 (65.8383, -0.4215)
  point P79 (61.5178, -28.1006)
  point P80 (-21.596, -25.9046)
  point P81 (-29.5518, -24.7156)
  point P82 (-32.5518, -18.4706)
  point P83 (32.8968, -28.1702)
  point P84 (47.8031, -29.0245)
  point P85 (20.1554, -30.2247)
  point P86 (20.0253, -27.2275)
  point P87 (47.673, -26.0274)
  point P88 (63.2105, 3.4664)
  point P89 (63.4275, 3.5864)
  point P90 (37.4913, -9.512)
  point P91 (62.8383, -7.2471)
  point P92 (62.8383, -1.6311)
  dimension "d294" = 3
  dimension "d297" = 5
  dimension "d316" = 16.005
  dimension "d269" = 3
  dimension "d271" = 5.5
  dimension "d274" = 3
  dimension "d275" = 3
  dimension "d276" = 3
  dimension "d277" = 3
  dimension "d278" = 3
  dimension "d279" = 10
  dimension "d280" = 3
  dimension "d281" = 3
  dimension "d282" = 3
  dimension "d283" = 1.5
  dimension "d285" = 3
  dimension "d286" = 3
  dimension "d287" = 3
  dimension "d288" = 3
  dimension "d289" = 3
  dimension "d290" = 3
  dimension "d291" = 3
  dimension "d292" = 3
  dimension "d295" = 2.1
  dimension "d296" = 2.1
  dimension "d301" = 4
  dimension "d302" = 6
  dimension "d303" = 3
  dimension "d304" = 3
  dimension "d307" = 3
  constraints: 136 end point, 54 point on circle, 46 tangent, 35 centre point, 13 parallel, 11 midpoint, 3 point on line, 1 vertical, 41 other
  measures "d269" distance between parallel lines of L8 L16
  measures "d271" radial gap between concentric circles of A13 A20
  measures "d274" radial gap between concentric circles of A8 A22
  measures "d275" radial gap between concentric circles of A11 A23
  measures "d276" radial gap between concentric circles of A10 A24
  measures "d277" radial gap between concentric circles of A7 A25
  measures "d278" diameter of A6
  measures "d279" distance of L29.end L30.end
  measures "d280" diameter of A28
  measures "d281" diameter of A30
  measures "d282" diameter of A34
  measures "d283" radius of A32
  measures "d285" diameter of A37
  measures "d286" diameter of A39
  measures "d287" radial gap between concentric circles of A9 A40
  measures "d288" diameter of A42
  measures "d289" diameter of A44
  measures "d290" diameter of A46
  measures "d291" distance between parallel lines of L56 L66
  measures "d292" distance between parallel lines of L55 L67
  measures "d295" diameter of A48
  measures "d296" diameter of A49
  measures "d301" diameter of A0
  measures "d304" distance between parallel lines of L68 L69
  measures "d307" diameter of A54
extrude "押し出し11" cut sketch "スケッチ13" against normal blind 3 contours A51 L69 A52 L41 A23 L39 | L64 L61 A44 L31 A50 L28 A51 | L38 A23 L61 L65 A51 | A50 | A51 L9 L8 L70 L68 L16 L28 | L28 L16 L68 A51 | L42 A52 L53 L50 A22 L44 A23 | L62 A23 L59 A25 A49 L26 A18 L32 L31 | L45 A22 L48 A24 L73 A23 | A23 L72 A24 L66 L21 L22 A26 A47 L35 L34 A17 L26 A48 A25 L58 | L17 A20 L50 L54 A52 | L51 L53 A21 A40 L67 A24 L47 A22 | A49 | L18 A21 L54 L51 A20 | L73 L48 A33 L72 A10 | A10 L48 L73 | A10 L47 A54 L73 L48 | L72 A33 L47 A10 | L73 A54 A33 L48 | A48 | A21 A9 | A9 A21 | L6 L14 L56 L21 L20 L55 | L55 L20 L21 L56 | A47
fillet "フィレット2" radius 1.05 64 edges at (23.1806, 30.9304, 1.5) (-19.0518, -55.4706, 1.5) (-29.5518, -24.7156, 1.5) (-21.596, -25.9046, 1.5) (-9.0325, -45.6326, 1.5) (-15.3311, -55.4706, 1.5) (-9.5518, -59.2398, 1.5) (13.3817, -37.8486, 1.5) (5.6941, -36.2112, 1.5) (19.383, -51.676, 1.5) (2.2911, -28.019, 1.5) (3.6677, -33.999, 1.5) (-6.7862, -43.575, 1.5) (-19.0656, -24.2931, 1.5) (-17.4474, -22.1485, 1.5) (-22.3223, -10.7876, 1.5) (-16.5922, -19.273, 1.5) (6.6325, -21.3707, 1.5) (3.1463, -25.1435, 1.5) (-7.025, -0.022, 1.5) (1.0695, -6.9431, 1.5) (19.201, -24.9423, 1.5) (16.1337, -36.6542, 1.5) (9.4316, -20.2914, 1.5) (17.3877, -22.5523, 1.5) (3.8686, -5.8638, 1.5) (7.0194, -0.2801, 1.5) (2.0091, 6.7316, 1.5) (6.4962, 2.6739, 1.5) (30.0511, 21.8718, 1.5) (23.3941, 26.9995, 1.5) (55.5088, 3.5636, 1.5) (55.2677, 17.3531, 1.5) (51.4464, 10.6354, 1.5) (32.1115, 7.2109, 1.5) (33.3602, -1.6742, 1.5) (28.1043, -14.4219, 1.5) (32.5293, 4.2382, 1.5) (35.4852, 4.7617, 1.5) (33.0219, 22.2893, 1.5) (35.0674, 7.7344, 1.5) (38.0109, 29.5649, 1.5) (59.4071, -22.1705, 1.5) (50.5472, -21.5001, 1.5) (36.3311, -1.2567, 1.5) (43.6318, -15.1503, 1.5) (41.6027, -17.36, 1.5) (29.9176, -16.8119, 1.5) (48.5182, -23.7099, 1.5) (58.0085, -33.3261, 1.5) (56.6989, -47.1291, 1.5) (56.3303, -47.4852, 1.5) (56.3303, -50.8831, 1.5) (31.4482, -59.2199, 1.5) (29.3513, -59.4706, 1.5) (22.135, -50.4815, 1.5) (47.673, -26.0274, 1.5) (20.0253, -27.2275, 1.5) (20.1554, -30.2247, 1.5) (47.8031, -29.0245, 1.5) (51.9696, 7.6814, 1.5) (62.5647, -1.9413, 1.5) (64.3298, 4.8026, 1.5) (61.2364, 16.8045, 1.5)
sketch "スケッチ14" plane through (0, 0, 0) normal (0, 0, -1) x (-1, 0, 0)
  circle A0 centre (-30.5138, 29.3575) radius 2 projected
  circle A1 centre (24.5518, -18.4706) radius 2 projected
  circle A2 centre (-30.5138, 29.3575) radius 4
  circle A3 centre (24.5518, -18.4706) radius 4
  point P0 (0, 0)
  dimension "d308" = 8
  dimension "d309" = 8
  constraints: 2 centre point, 2 coincident
  measures "d308" diameter of A2
  measures "d309" diameter of A3
extrude "押し出し12" cut sketch "スケッチ14" against normal blind 0.5
equation "\"d40\" = d39"
equation "\"d41\" = d40"
